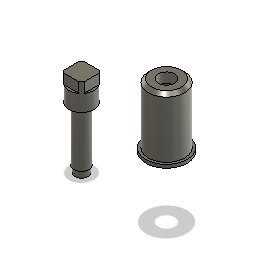
a2m0032_paper_roll_pin_ v7 (Autodesk Fusion 360 design; units mm, degrees)
Autodesk Fusion 360 part; units mm, degrees
sketch "Sketch1" plane through (0, 0, 0) normal (0, 1, 0) x (1, 0, 0) in component "SPINDLE"
  circle A0 centre (0, 0) radius 3.8
  line L0 (-3.05, 3.05) -> (3.05, 3.05)
  line L1 (3.05, 3.05) -> (3.05, -3.05)
  line L2 (3.05, -3.05) -> (-3.05, -3.05)
  line L3 (-3.05, -3.05) -> (-3.05, 3.05)
  line L4 (-3.05, 3.05) -> (3.05, -3.05) construction
  line L5 (3.05, 3.05) -> (-3.05, -3.05) construction
  circle A1 centre (0, 0) radius 2.3
  dimension "d3" = 7.6
  dimension "d4" = 6.1
  dimension "d5" = 6.1
  dimension "d6" = 4.6
  constraint horizontal L0
  constraint perpendicular L0 L1
  constraint parallel L0 L2
  constraint parallel L1 L3
  constraint coincident L4 A0.centre
  constraint coincident L5 A0.centre
  constraint coincident A0.centre A1.centre
  measures "d3" diameter of A0
  measures "d4" distance of L0.end L1.end
  measures "d5" distance of L1.end L2.end
  measures "d6" diameter of A1
sketch "Sketch2" plane through (0, 0, 0) normal (0, 1, 0) x (1, 0, 0) in component "DRUM"
  line L0 (25.6191, 10.852) -> (25.6191, -10.852) construction
  line L1 (12.1191, 0) -> (39.1191, 0) construction
  circle A0 centre (25.6191, 0) radius 6.2
  circle A1 centre (25.6191, 0) radius 5.45
  circle A2 centre (25.6191, 0) radius 2.45
  circle A3 centre (25.6191, 0) radius 3.9
  dimension "d7" = 12.4
  dimension "d8" = 10.9
  dimension "d9" = 4.9
  dimension "d10" = 7.8
  constraint vertical L0
  constraint horizontal L1
  constraint midpoint L0 L1
  constraint horizontal L1.start origin
  constraint midpoint L0 A0.centre
  constraint concentric A0 A1
  constraint concentric A0 A2
  constraint concentric A0 A3
  measures "d7" diameter of A0
  measures "d8" diameter of A1
  measures "d9" diameter of A2
  measures "d10" diameter of A3
extrude "Extrude1" add sketch "Sketch1" against normal blind 18.4 contours A1 makes body 1 in component "SPINDLE"
extrude "Extrude2" add sketch "Sketch1" along normal blind 5 contours A0 L1 | A0 L0 L1 L2 L3 | A0 L0 | A0 L2 | A0 L3 | A1 bodies 1 in component "SPINDLE"
extrude "Extrude3" add sketch "Sketch1" along normal blind 8 contours A0 L0 L1 L2 L3 | A1 bodies 1 in component "SPINDLE"
extrude "Extrude1'" add sketch "Sketch2" along normal blind 19 separate body contours A1 | A3 makes body 2 in component "DRUM"
extrude "Extrude2'" add sketch "Sketch2" along normal blind 1 contours A0 bodies 2 in component "DRUM"
extrude "Extrude3'" cut sketch "Sketch2" along normal blind 16 contours A3 bodies 2 in component "DRUM"
chamfer "Chamfer1" distance 1 angle 45 1 edges at (20.538, 19, 1.9708) on bodies 2 in component "DRUM"
sketch "Sketch3" plane through (0, -18.4, 0) normal (0, -1, 0) x (1, 0, 0)
  circle A0 centre (0, 0) radius 2.3
  circle A1 centre (0, 0) radius 2
  dimension "d24" = 4
  constraint concentric A0 A1
  measures "d24" diameter of A1
extrude "Extrude4" cut sketch "Sketch3" against normal blind 2 bodies 1 in component "SPINDLE"
component "SPINDLE" placed x (1, 0, 0) y (0, 1, 0) z (0, 0, 1) at (0, 0, 0)
component "DRUM" placed x (1, 0, 0) y (0, 1, 0) z (0, 0, 1) at (0, 0, 0)
equation "d5 = d4"
